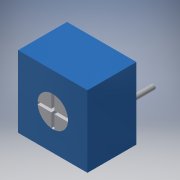
# Autodesk Inventor part: Poti
Saved by Autodesk Inventor 2019 (Build 230136000, 136)
## iProperties
Created: 2019-06-05
Part Number: Poti
Material: PBT-Kunststoff
Document SubType Name: Modeling
Designer: manue
Density: 1.31 g/cm^3
Appearance: Cyan
Author: manue
Autodesk Inventor part; units mm, degrees
ref_plane "YZ Plane" through (0, 0, 0) normal (1, 0, 0) x (0, 1, 0)
ref_plane "XZ Plane" through (0, 0, 0) normal (0, 1, 0) x (-1, 0, 0)
ref_plane "XY Plane" through (0, 0, 0) normal (0, 0, 1) x (1, 0, 0)
sketch "Skizze1" plane through (0, 0, 0) normal (0, 0, 1) x (1, 0, 0)
  line L0 (0, 0) -> (6.8, 0)
  line L1 (6.8, 0) -> (6.8, 7)
  line L2 (6.8, 7) -> (0, 7)
  line L3 (0, 7) -> (0, 0)
  dimension "d0" = 6.8
  dimension "d1" = 7
  constraints: 8 end point, 2 parallel, 1 horizontal, 1 perpendicular
  measures "d0" distance of L2.end L1.end
  measures "d1" distance of L1.end L0.end
extrude "Extrusion1" add sketch "Skizze1" along normal blind 4.8
sketch "Skizze2" plane through (0, 0, 4.8) normal (0, 0, 1) x (1, 0, 0)
  line L0 (0, 0) -> (6.8, 0) construction
  line L1 (6.8, 0) -> (6.8, 7) construction
  line L2 (6.8, 7) -> (0, 7) construction
  line L3 (0, 7) -> (0, 0) construction
  circle A0 centre (3.4, 3.5) radius 1.5
  point P0 (0, 3.5)
  point P1 (3.4, 7)
  dimension "d4" = 3
  constraints: 2 midpoint, 1 centre point, 1 horizontal alignment, 1 vertical alignment
  measures "d4" diameter of A0
extrude "Extrusion2" cut sketch "Skizze2" against normal blind 0.01
sketch "Skizze3" plane through (3.4, 3.5, 4.79) normal (0, 0, 1) x (1, 0, 0)
  line L0 (-0.15, 1.4925) -> (0.15, 1.4925)
  line L1 (0.15, -1.4925) -> (-0.15, -1.4925)
  line L2 (1.4925, 0.15) -> (1.4925, -0.15)
  line L3 (-1.4925, -0.15) -> (-1.4925, 0.15)
  line L4 (-1.4925, 0.15) -> (-0.15, 0.15)
  line L5 (0.15, 0.15) -> (1.4925, 0.15)
  line L6 (0.15, 1.4925) -> (0.15, 0.15)
  line L7 (0.15, -0.15) -> (0.15, -1.4925)
  line L8 (-0.15, -1.4925) -> (-0.15, -0.15)
  line L9 (-0.15, 0.15) -> (-0.15, 1.4925)
  line L10 (1.4925, -0.15) -> (0.15, -0.15)
  line L11 (-0.15, -0.15) -> (-1.4925, -0.15)
  line L12 (0, 1.4925) -> (0, -1.4925) construction
  line L13 (-1.4925, 0) -> (1.4925, 0) construction
  circle A0 centre (0, 0) radius 1.5 construction
  point P0 (-3.4, -3.5)
  dimension "d7" = 0.3
  constraints: 28 end point, 10 parallel, 5 perpendicular, 4 collinear, 4 equal length, 4 midpoint, 3 horizontal, 3 point on circle
  measures "d7" distance between parallel lines of L6 L9
extrude "Extrusion3" cut sketch "Skizze3" against normal blind 1.5
sketch "Skizze4" plane through (0, 0, 0) normal (0, 0, -1) x (-1, 0, 0)
  circle A0 centre (-0.86, 3.22) radius 0.25
  circle A1 centre (-5.94, 3.22) radius 0.25
  circle A2 centre (-3.4, 0.68) radius 0.25
  line L0 (0, 0) -> (-6.8, 0) construction
  line L1 (-3.4, 0) -> (-3.4, 7) construction
  line L2 (-6.8, 7) -> (0, 7) construction
  dimension "d10" = 0.5
  dimension "d11" = 5.08
  dimension "d12" = 2.54
  dimension "d13" = 0.68
  constraints: 3 centre point, 2 end point, 2 equal radius, 2 midpoint, 1 horizontal alignment, 1 point on line, 1 symmetric about line
  measures "d10" diameter of A0
  measures "d11" distance of A1.centre A0.centre
  measures "d12" horizontal distance of A2.centre A1.centre
  measures "d13" distance from line of L0 A2.centre
extrude "Extrusion4" add sketch "Skizze4" along normal blind 2.5
